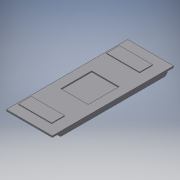
# Autodesk Inventor part: Button
Saved by Autodesk Inventor 2016 SP2 (Build 200236200, 236)
## iProperties
Created: 2018-06-26
Part Number: Button
Material: Generisch
Document SubType Name: Modeling
Designer: Nils
Density: 1 g/cm^3
Appearance: Vorgabe
Author: Nils
Autodesk Inventor part; units mm, degrees
ref_plane "YZ Plane" through (0, 0, 0) normal (1, 0, 0) x (0, 1, 0)
ref_plane "XZ Plane" through (0, 0, 0) normal (0, 1, 0) x (-1, 0, 0)
ref_plane "XY Plane" through (0, 0, 0) normal (0, 0, 1) x (1, 0, 0)
sketch "Skizze1" plane through (0, 0, 0) normal (0, 0, 1) x (1, 0, 0)
  arc A0 (-10.6401, 53.1217) -> (-12.6401, 51.1217) centre (-10.6401, 51.1217) ccw construction
  line L0 (-12.6401, 51.1217) -> (-12.6401, -3.8783) construction
  arc A1 (-12.6401, -3.8783) -> (-10.6401, -5.8783) centre (-10.6401, -3.8783) ccw construction
  line L1 (-10.6401, -5.8783) -> (35.6599, -5.8783) construction
  arc A2 (35.6599, -5.8783) -> (37.6599, -3.8783) centre (35.6599, -3.8783) ccw construction
  line L2 (37.6599, -3.8783) -> (37.6599, 51.1217) construction
  arc A3 (37.6599, 51.1217) -> (35.6599, 53.1217) centre (35.6599, 51.1217) ccw construction
  line L3 (35.6599, 53.1217) -> (-10.6401, 53.1217) construction
  arc A4 (-24.2401, -8.4283) -> (-19.5401, -13.1283) centre (-19.5401, -8.4283) ccw construction
  line L4 (-24.2401, 55.6717) -> (-24.2401, -8.4283) construction
  arc A5 (-19.5401, 60.3717) -> (-24.2401, 55.6717) centre (-19.5401, 55.6717) ccw construction
  line L5 (44.5599, 60.3717) -> (-19.5401, 60.3717) construction
  arc A6 (49.2599, 55.6717) -> (44.5599, 60.3717) centre (44.5599, 55.6717) ccw construction
  line L6 (49.2599, -8.4283) -> (49.2599, 55.6717) construction
  arc A7 (44.5599, -13.1283) -> (49.2599, -8.4283) centre (44.5599, -8.4283) ccw construction
  line L7 (-19.5401, -13.1283) -> (44.5599, -13.1283) construction
  line L8 (35.6599, -5.7783) -> (-10.6401, -5.7783)
  arc A8 (-12.5401, -3.8783) -> (-10.6401, -5.7783) centre (-10.6401, -3.8783) ccw
  line L9 (-12.5401, -3.8783) -> (-12.5401, 51.1217)
  arc A9 (-10.6401, 53.0217) -> (-12.5401, 51.1217) centre (-10.6401, 51.1217) ccw
  line L10 (-10.6401, 53.0217) -> (35.6599, 53.0217)
  arc A10 (37.5599, 51.1217) -> (35.6599, 53.0217) centre (35.6599, 51.1217) ccw
  line L11 (37.5599, 51.1217) -> (37.5599, -3.8783)
  arc A11 (35.6599, -5.7783) -> (37.5599, -3.8783) centre (35.6599, -3.8783) ccw
  line L12 (12.5099, -5.7783) -> (12.5099, 53.0217) construction
  line L13 (12.3599, 53.0217) -> (12.3599, -5.7783)
  point P0 (0, 0)
  dimension "d0" = 0.1
  dimension "d1" = 24.9
  constraints: 12 end point, 8 point on circle, 4 centre point, 2 midpoint, 2 point on line, 1 perpendicular, 7 other
  measures "d0" distance between parallel lines of L1 L8
  measures "d1" distance between parallel lines of L13 L9
extrude "Extrusion1" add sketch "Skizze1" along normal blind 1.8 contours L8 A8 L9 A9 L10 L13
sketch "Skizze2" plane through (0, 0, 1.8) normal (0, 0, 1) x (1, 0, 0)
  line L0 (12.3599, 56.5217) -> (-12.5401, 56.5217)
  line L1 (-12.5401, 56.5217) -> (-12.5401, -9.2783)
  line L2 (-12.5401, -9.2783) -> (12.3599, -9.2783)
  line L3 (12.3599, -9.2783) -> (12.3599, 56.5217)
  line L4 (-10.6401, -5.7783) -> (12.3599, -5.7783) projected
  line L5 (12.3599, 53.0217) -> (-10.6401, 53.0217) projected
  line L6 (12.3599, -5.7783) -> (12.3599, 53.0217) projected
  line L7 (-12.5401, 51.1217) -> (-12.5401, -3.8783) projected
  point P0 (0, 0)
  dimension "d4" = 3.5
  dimension "d5" = 3.5
  constraints: 8 end point, 2 collinear, 2 parallel, 1 horizontal, 1 perpendicular
  measures "d4" distance between parallel lines of L2 L4
  measures "d5" distance between parallel lines of L0 L5
extrude "Extrusion2" add sketch "Skizze2" along normal blind 0.8
sketch "Skizze3" plane through (0, 0, 2.6) normal (0, 0, 1) x (1, 0, 0)
  line L0 (-11.5401, 51.0217) -> (6.4599, 51.0217)
  line L1 (6.4599, 51.0217) -> (6.4599, 44.0217)
  line L2 (6.4599, 44.0217) -> (-11.5401, 44.0217)
  line L3 (-11.5401, 44.0217) -> (-11.5401, 51.0217)
  line L4 (-11.5401, 3.2217) -> (6.4599, 3.2217)
  line L5 (6.4599, 3.2217) -> (6.4599, -3.7783)
  line L6 (6.4599, -3.7783) -> (-11.5401, -3.7783)
  line L7 (-11.5401, -3.7783) -> (-11.5401, 3.2217)
  line L8 (12.3599, 56.5217) -> (-12.5401, 56.5217) projected
  line L9 (-12.5401, -9.2783) -> (12.3599, -9.2783) projected
  line L10 (-12.5401, -3.8783) -> (-12.5401, -9.2783) projected
  point P0 (0, 0)
  dimension "d8" = 18
  dimension "d9" = 18
  dimension "d10" = 7
  dimension "d11" = 7
  dimension "d12" = 5.5
  dimension "d13" = 5.5
  dimension "d14" = 1
  constraints: 16 end point, 4 parallel, 2 horizontal, 2 perpendicular, 1 point on line
  measures "d8" distance of L1.end L2.end
  measures "d9" distance of L4.start L4.end
  measures "d10" distance of L0.end L1.end
  measures "d11" distance of L4.end L5.end
  measures "d12" distance between parallel lines of L8 L0
  measures "d13" distance between parallel lines of L9 L6
  measures "d14" distance between parallel lines of L10 L7
extrude "Extrusion3" add sketch "Skizze3" along normal blind 0.4
chamfer "Fase1" distance 1 angle 45 5 edges at (0.8599, 53.0217, 0) (-11.9836, 52.4652, 0) (-12.5401, 23.6217, 0) (-11.9836, -5.2218, 0) (0.8599, -5.7783, 0)
sketch "Skizze4" plane through (0, 0, 0) normal (0, 0, -1) x (-1, 0, 0)
  line L0 (10.6401, -4.7783) -> (-12.3599, -4.7783) construction
  line L1 (-12.3599, 52.0217) -> (10.6401, 52.0217) construction
  line L2 (-6.9071, 11.4129) -> (4.4149, 11.4129) construction
  line L3 (4.4149, 11.4129) -> (4.4149, 1.8512) construction
  line L4 (4.4149, 1.8512) -> (-6.9071, 1.8512) construction
  line L5 (-6.9071, 1.8512) -> (-6.9071, 11.4129) construction
  line L6 (-3.8878, 41.1888) -> (4.1122, 41.1888) construction
  line L7 (4.1122, 41.1888) -> (4.1122, 36.9997) construction
  line L8 (4.1122, 36.9997) -> (-3.8878, 36.9997) construction
  line L9 (-3.8878, 36.9997) -> (-3.8878, 41.1888) construction
  line L10 (11.5401, 51.1217) -> (11.5401, -3.8783) construction
  line L11 (11.5401, 40.0217) -> (-12.3599, 40.0217) construction
  line L12 (11.5401, 7.2217) -> (-12.3599, 7.2217) construction
  line L13 (-12.3599, -4.7783) -> (-12.3599, 52.0217) construction
  line L14 (-0.8599, -4.7783) -> (-0.8599, 52.0217) construction
  line L15 (3.8385, 6.0547) -> (-0.2263, 6.0547)
  line L16 (-0.2263, 6.0547) -> (-0.2263, 1.9899)
  line L17 (-0.2263, 1.9899) -> (-1.5683, 1.9899)
  line L18 (-1.5683, 1.9899) -> (-1.5683, 6.0547)
  line L19 (-1.5683, 6.0547) -> (-5.6332, 6.0547)
  line L20 (-5.6332, 6.0547) -> (-5.6332, 7.348)
  line L21 (-5.6332, 7.348) -> (-1.5683, 7.348)
  line L22 (-1.5683, 7.348) -> (-1.5683, 11.4129)
  line L23 (-1.5683, 11.4129) -> (-0.2263, 11.4129)
  line L24 (-0.2263, 11.4129) -> (-0.2263, 7.348)
  line L25 (-0.2263, 7.348) -> (3.8385, 7.348)
  line L26 (3.8385, 7.348) -> (3.8385, 6.0547)
  line L27 (1.3829, 39.7301) -> (-3.1585, 39.7301)
  line L28 (-3.1585, 39.7301) -> (-3.1585, 41.1888)
  line L29 (-3.1585, 41.1888) -> (1.3829, 41.1888)
  line L30 (1.3829, 41.1888) -> (1.3829, 39.7301)
  point P0 (0, 0)
  dimension "d20" = 12
  dimension "d21" = 12
  constraints: 6 end point, 3 point on line, 2 horizontal, 2 midpoint, 4 other
  measures "d20" distance between parallel lines of L1 L11
  measures "d21" distance between parallel lines of L12 L0
extrude "Extrusion4" cut sketch "Skizze4" against normal blind 0.4
sketch "Skizze5" plane through (0, 0, 2.6) normal (0, 0, 1) x (1, 0, 0)
  line L0 (7.3599, 32.0217) -> (-7.5401, 32.0217)
  line L1 (-7.5401, 32.0217) -> (-7.5401, 15.2217)
  line L2 (-7.5401, 15.2217) -> (7.3599, 15.2217)
  line L3 (7.3599, 15.2217) -> (7.3599, 32.0217)
  line L4 (6.4599, 44.0217) -> (-11.5401, 44.0217) projected
  line L5 (6.4599, 3.2217) -> (-11.5401, 3.2217) projected
  line L6 (-12.5401, 56.5217) -> (-12.5401, -9.2783) projected
  line L7 (12.3599, -9.2783) -> (12.3599, 56.5217) projected
  point P0 (0, 0)
  dimension "d24" = 12
  dimension "d25" = 12
  dimension "d26" = 5
  dimension "d27" = 5
  constraints: 8 end point, 2 parallel, 1 horizontal, 1 perpendicular
  measures "d24" distance between parallel lines of L4 L0
  measures "d25" distance between parallel lines of L2 L5
  measures "d26" distance between parallel lines of L6 L1
  measures "d27" distance between parallel lines of L7 L3
extrude "Extrusion5" cut sketch "Skizze5" against normal blind 0.6
equation "\"d5\" = d4"
equation "\"d9\" = d8"
equation "\"d13\" = d12"
